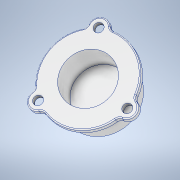
# Autodesk Inventor part: EndCap
Saved by Autodesk Inventor 2020.2 (Build 242292000, 292)
## iProperties
RuleStatus: InUse
Created: 2020-07-14
Part Number: EndCap
Material: Aluminum 6061
Document SubType Name: Modeling
Designer: holecep
Density: 2.7 g/cm^3
Appearance: Aluminum - Flat
Mass: 169.065 g
Surface Area: 207.044 cm^2
Volume: 62.6167 cm^3
Author: holecep
Autodesk Inventor part; units mm, degrees
ref_plane "YZ Plane" through (0, 0, 0) normal (1, 0, 0) x (0, 1, 0)
ref_plane "XZ Plane" through (0, 0, 0) normal (0, 1, 0) x (-1, 0, 0)
ref_plane "XY Plane" through (0, 0, 0) normal (0, 0, 1) x (1, 0, 0)
sketch "Sketch1" plane through (0, 0, 0) normal (0, 1, 0) x (-1, 0, 0)
  circle A0 centre (0, 0) radius 38
  dimension "d0" = 76
  constraints: 1 centre point, 1 coincident
  measures "d0" diameter of A0
extrude "Extrusion1" add sketch "Sketch1" along normal blind 5
sketch "Sketch2" plane through (0, 0, 0) normal (0, -1, 0) x (1, 0, 0)
  circle A0 centre (0, 0) radius 38 projected
  circle A1 centre (0, 38) radius 8
  circle A2 centre (0, 38) radius 4
  point P0 (-3.9945, 37.7895)
  point P1 (3.9945, 37.7895)
  point P2 (7.9556, 37.1579)
  point P3 (-7.9556, 37.1579)
  dimension "d3" = 8
  dimension "d4" = 16
  constraints: 2 centre point, 1 coincident, 2 other
  measures "d3" diameter of A2
  measures "d4" diameter of A1
extrude "Extrusion2" add sketch "Sketch2" against normal blind 5 contours A0 A2 A1 | A2 A0 picked at (6.1003, 40.5657) picked at (-0.1554, 36.6601)
sketch "Sketch3" plane through (0, 0, 0) normal (0, -1, 0) x (1, 0, 0)
  circle A0 centre (0, 38) radius 4 projected
  point P0 (0, 0)
extrude "Extrusion3" cut sketch "Sketch3" against normal up to next
sketch "Sketch4" plane through (0, 5, 0) normal (0, 1, 0) x (1, 0, 0)
  circle A0 centre (0, 0) radius 30
  dimension "d9" = 60
  constraints: 1 centre point, 1 coincident
  measures "d9" diameter of A0
extrude "Extrusion4" add sketch "Sketch4" along normal blind 30
sketch "Sketch5" plane through (0, 0, 0) normal (0, -1, 0) x (1, 0, 0)
  circle A0 centre (0, 0) radius 22
  circle A1 centre (0, 0) radius 30 projected
  dimension "d12" = 8
  constraints: 1 centre point, 1 coincident
  measures "d12" radial gap between concentric circles of A0 A1
extrude "Extrusion5" cut sketch "Sketch5" against normal blind 30 contours A0
fillet "Fillet1" radius 5 2 edges at (-7.9556, 2.5, 37.1579) (7.9556, 2.5, 37.1579)
pattern_circular "Circular Pattern1" count 3 over 360 about axis through (0, 0, 0) along (0, 1, 0) of "Extrusion2", "Fillet1", "Extrusion3"
fillet "Fillet2" radius 1 12 edges at (0, 0, 46) (8.9892, 0, 37.6715) (32.909, 0, 19) (37.1191, 0, -11.0508) (39.8372, 0, -23) (28.1298, 0, -26.6207) (0, 0, -38) (-28.1298, 0, -26.6207) (-39.8372, 0, -23) (-37.1191, 0, -11.0508) (-32.909, 0, 19) (-8.9892, 0, 37.6715)
chamfer "Chamfer1" distance 1 angle 45 1 edges at (-30, 35, 0)
equation "\"d0\" = d9 + 2 * BoltDiameter"
equation "\"d3\" = BoltDiameter"
equation "\"d4\" = 2 * d3"
equation "\"d9\" = Diameter"
equation "\"d10\" = Depth"
equation "\"d12\" = d3"
equation "\"d13\" = d10"
equation "\"Diameter\" = 60"
equation "\"BoltDiameter\" = 8"
equation "\"Depth\" = 30"
body "Solid1"
